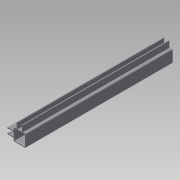
# Autodesk Inventor part: 9030
Saved by Autodesk Inventor 2013 (Build 170138000, 138)
## iProperties
Created: 2014-04-23
Part Number: 9030
Material: Generic
Document SubType Name: Modeling
Density: 1 g/cm^3
Vendor: 80/20 Inc.
Engineer: Ross Bowman
Designer: Ross Bowman
Catalog Web Link: 8020.net
Company: 80/20 Inc.
Author: Ross Bowman
Keywords: 80/20 , 8020 , T-Slot , Extrusion
Material: 6105-T5 Aluminum
Autodesk Inventor part; units mm, degrees
ref_plane "YZ Plane" through (0, 0, 0) normal (1, 0, 0) x (0, 1, 0)
ref_plane "XZ Plane" through (0, 0, 0) normal (0, 1, 0) x (-1, 0, 0)
ref_plane "XY Plane" through (0, 0, 0) normal (0, 0, 1) x (1, 0, 0)
sketch "Sketch1" plane through (0, 0, 0) normal (0, 0, 1) x (1, 0, 0)
  line L0 (-9.652, -11.176) -> (9.652, -11.176)
  arc A0 (-11.176, -9.652) -> (-9.652, -11.176) centre (-9.652, -9.652) ccw
  line L1 (-11.176, 9.652) -> (-11.176, -9.652)
  arc A1 (-9.652, 11.176) -> (-11.176, 9.652) centre (-9.652, 9.652) ccw
  line L2 (9.652, 11.176) -> (-9.652, 11.176)
  arc A2 (11.176, 9.652) -> (9.652, 11.176) centre (9.652, 9.652) ccw
  line L3 (11.176, -9.652) -> (11.176, 9.652)
  arc A3 (9.652, -11.176) -> (11.176, -9.652) centre (9.652, -9.652) ccw
  arc A4 (-6.731, 12.7) -> (-6.35, 13.081) centre (-6.731, 13.081) ccw
  line L4 (-6.731, 12.7) -> (-10.5918, 12.7)
  arc A5 (-10.5918, 12.7) -> (-12.7, 10.5918) centre (-10.5918, 10.5918) ccw
  line L5 (-12.7, 10.5918) -> (-12.7, 6.731)
  arc A6 (-13.081, 6.35) -> (-12.7, 6.731) centre (-13.081, 6.731) ccw
  line L6 (-13.081, 6.35) -> (-25.019, 6.35)
  arc A7 (-25.019, 6.35) -> (-25.4, 5.969) centre (-25.019, 5.969) ccw
  line L7 (-25.4, 5.969) -> (-25.4, 4.826)
  arc A8 (-25.4, 4.826) -> (-24.638, 4.064) centre (-24.638, 4.826) ccw
  line L8 (-24.638, 4.064) -> (-23.0632, 4.064)
  arc A9 (-23.0632, 4.064) -> (-22.6822, 4.445) centre (-23.0632, 4.445) ccw
  arc A10 (-22.3012, 4.826) -> (-22.6822, 4.445) centre (-22.3012, 4.445) ccw
  line L9 (-22.3012, 4.826) -> (-13.081, 4.826)
  arc A11 (-12.7, 4.445) -> (-13.081, 4.826) centre (-13.081, 4.445) ccw
  line L10 (-12.7, 4.445) -> (-12.7, -4.445)
  arc A12 (-13.081, -4.826) -> (-12.7, -4.445) centre (-13.081, -4.445) ccw
  line L11 (-13.081, -4.826) -> (-22.3012, -4.826)
  arc A13 (-22.6822, -4.445) -> (-22.3012, -4.826) centre (-22.3012, -4.445) ccw
  arc A14 (-22.6822, -4.445) -> (-23.0632, -4.064) centre (-23.0632, -4.445) ccw
  line L12 (-23.0632, -4.064) -> (-24.638, -4.064)
  arc A15 (-24.638, -4.064) -> (-25.4, -4.826) centre (-24.638, -4.826) ccw
  line L13 (-25.4, -4.826) -> (-25.4, -5.969)
  arc A16 (-25.4, -5.969) -> (-25.019, -6.35) centre (-25.019, -5.969) ccw
  line L14 (-25.019, -6.35) -> (-13.081, -6.35)
  arc A17 (-12.7, -6.731) -> (-13.081, -6.35) centre (-13.081, -6.731) ccw
  line L15 (-12.7, -6.731) -> (-12.7, -10.5918)
  arc A18 (-12.7, -10.5918) -> (-10.5918, -12.7) centre (-10.5918, -10.5918) ccw
  line L16 (-10.5918, -12.7) -> (10.5918, -12.7)
  arc A19 (10.5918, -12.7) -> (12.7, -10.5918) centre (10.5918, -10.5918) ccw
  line L17 (12.7, -10.5918) -> (12.7, 10.5918)
  arc A20 (12.7, 10.5918) -> (10.5918, 12.7) centre (10.5918, 10.5918) ccw
  line L18 (10.5918, 12.7) -> (6.731, 12.7)
  arc A21 (6.35, 13.081) -> (6.731, 12.7) centre (6.731, 13.081) ccw
  line L19 (6.35, 13.081) -> (6.35, 25.019)
  arc A22 (6.35, 25.019) -> (5.969, 25.4) centre (5.969, 25.019) ccw
  line L20 (5.969, 25.4) -> (4.826, 25.4)
  arc A23 (4.826, 25.4) -> (4.064, 24.638) centre (4.826, 24.638) ccw
  line L21 (4.064, 24.638) -> (4.064, 23.0632)
  arc A24 (4.064, 23.0632) -> (4.445, 22.6822) centre (4.445, 23.0632) ccw
  arc A25 (4.826, 22.3012) -> (4.445, 22.6822) centre (4.445, 22.3012) ccw
  line L22 (4.826, 22.3012) -> (4.826, 13.081)
  arc A26 (4.445, 12.7) -> (4.826, 13.081) centre (4.445, 13.081) ccw
  line L23 (4.445, 12.7) -> (-4.445, 12.7)
  arc A27 (-4.826, 13.081) -> (-4.445, 12.7) centre (-4.445, 13.081) ccw
  line L24 (-4.826, 13.081) -> (-4.826, 22.3012)
  arc A28 (-4.445, 22.6822) -> (-4.826, 22.3012) centre (-4.445, 22.3012) ccw
  arc A29 (-4.445, 22.6822) -> (-4.064, 23.0632) centre (-4.445, 23.0632) ccw
  line L25 (-4.064, 23.0632) -> (-4.064, 24.638)
  arc A30 (-4.064, 24.638) -> (-4.826, 25.4) centre (-4.826, 24.638) ccw
  line L26 (-4.826, 25.4) -> (-5.969, 25.4)
  arc A31 (-5.969, 25.4) -> (-6.35, 25.019) centre (-5.969, 25.019) ccw
  line L27 (-6.35, 25.019) -> (-6.35, 13.081)
  point P0 (0, 0)
  constraints: 64 point on circle, 60 tangent, 56 end point, 32 centre point, 20 parallel, 6 collinear, 1 horizontal, 1 vertical
extrude "Extrusion1" add sketch "Sketch1" against normal blind 304.8
body "Solid1"
